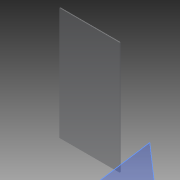
# Autodesk Inventor part: Collector Side
Saved by Autodesk Inventor 2014 (Build 180170000, 170)
## iProperties
Created: 2014-01-23
Part Number: Collector Side
Material: Polycarbonate, Clear
Document SubType Name: Modeling
Designer: Andrew Toennies
Mass: 275.303 g
Surface Area: 1480.64 cm^2
Volume: 229.419 cm^3
Density: 1.2 g/cm^3
Appearance: Polycarbonate - Clear
Author: Andrew Toennies
Autodesk Inventor part; units mm, degrees
ref_plane "YZ Plane" through (0, 0, 0) normal (1, 0, 0) x (0, 1, 0)
ref_plane "XZ Plane" through (0, 0, 0) normal (0, 1, 0) x (-1, 0, 0)
ref_plane "XY Plane" through (0, 0, 0) normal (0, 0, 1) x (1, 0, 0)
sketch "Sketch1" plane through (0, 0, 0) normal (0, 0, 1) x (1, 0, 0)
  line L0 (0, 0) -> (203.2, 0)
  line L1 (203.2, 381) -> (0, 381)
  line L2 (203.2, 352.425) -> (177.8, 352.425)
  line L3 (177.8, 352.425) -> (177.8, 323.85)
  line L4 (177.8, 323.85) -> (146.05, 323.85)
  line L5 (146.05, 323.85) -> (146.05, 285.75)
  line L6 (146.05, 285.75) -> (177.8, 285.75)
  line L7 (177.8, 285.75) -> (177.8, 206.375)
  line L8 (177.8, 206.375) -> (203.2, 206.375)
  line L9 (0, 352.425) -> (25.4, 352.425)
  line L10 (25.4, 352.425) -> (25.4, 323.85)
  line L11 (25.4, 323.85) -> (57.15, 323.85)
  line L12 (57.15, 323.85) -> (57.15, 285.75)
  line L13 (57.15, 285.75) -> (25.4, 285.75)
  line L14 (25.4, 285.75) -> (25.4, 257.175)
  line L15 (25.4, 257.175) -> (0, 257.175)
  line L16 (203.2, 0) -> (203.2, 206.375)
  line L17 (203.2, 352.425) -> (203.2, 381)
  line L18 (0, 381) -> (0, 352.425)
  line L19 (0, 257.175) -> (0, 0)
  dimension "d0" = 203.2
  dimension "d1" = 381
  dimension "d4" = 25.4
  dimension "d5" = 28.575
  dimension "d6" = 31.75
  dimension "d7" = 38.1
  dimension "d8" = 79.375
  dimension "d9" = 28.575
  dimension "d10" = 25.4
  dimension "d11" = 28.575
  dimension "d12" = 31.75
  dimension "d13" = 38.1
  dimension "d14" = 31.75
  dimension "d15" = 28.575
  dimension "d16" = 28.575
  constraints: 40 end point, 12 parallel, 10 perpendicular, 5 collinear, 1 horizontal
  measures "d0" distance of L1.start L1.end
  measures "d1" distance of L0.end L1.start
  measures "d4" distance of L2.start L2.end
  measures "d5" distance of L2.end L3.end
  measures "d6" distance of L3.end L4.end
  measures "d7" distance of L4.end L5.end
  measures "d8" distance of L6.end L7.end
  measures "d9" distance between parallel lines of L1 L2
  measures "d10" distance of L9.start L9.end
  measures "d11" distance of L9.end L10.end
  measures "d12" distance of L10.end L11.end
  measures "d13" distance of L11.end L12.end
  measures "d14" distance of L12.end L13.end
  measures "d15" distance of L13.end L14.end
  measures "d16" distance between parallel lines of L1 L9
extrude "Extrusion1" add sketch "Sketch1" along normal blind 3.175
body "Solid1"
